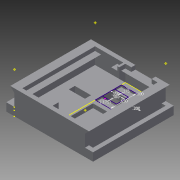
# Autodesk Inventor part: nano_enclosure_v3
Saved by Autodesk Inventor 2015 (Build 190159000, 159)
## iProperties
Created: 2015-03-02
Part Number: nano_enclosure_v3
Material: Generic
Document SubType Name: Modeling
Designer: Jeff
Density: 1 g/cm^3
Appearance: Default
Author: Jeff
Autodesk Inventor part; units mm, degrees
ref_plane "YZ Plane" through (0, 0, 0) normal (1, 0, 0) x (0, 1, 0)
ref_plane "XZ Plane" through (0, 0, 0) normal (0, 1, 0) x (-1, 0, 0)
ref_plane "XY Plane" through (0, 0, 0) normal (0, 0, 1) x (1, 0, 0)
sketch "Sketch2" plane through (0, 0, 0) normal (0, 0, 1) x (1, 0, 0)
  line L0 (0, 0) -> (44.45, 0)
  line L1 (44.45, 0) -> (44.45, 50.8)
  line L2 (44.45, 50.8) -> (0, 50.8)
  line L3 (0, 50.8) -> (0, 0)
  dimension "d0" = 50.8
  dimension "d1" = 44.45
  constraints: 8 end point, 2 parallel, 1 horizontal, 1 perpendicular
  measures "d0" distance of L0.end L1.end
  measures "d1" distance of L1.end L2.end
extrude "Extrusion1" add sketch "Sketch2" along normal blind 25.4
sketch "Sketch3" plane through (0, 0, 25.4) normal (0, 0, 1) x (1, 0, 0)
  line L0 (2.54, 2.54) -> (20.32, 2.54)
  line L1 (20.32, 2.54) -> (20.32, 48.26)
  line L2 (20.32, 48.26) -> (2.54, 48.26)
  line L3 (2.54, 48.26) -> (2.54, 2.54)
  line L4 (0, 0) -> (44.45, 0) projected
  line L5 (0, 50.8) -> (0, 0) projected
  line L6 (44.45, 50.8) -> (0, 50.8) projected
  line L7 (21.59, 2.54) -> (41.91, 2.54)
  line L8 (41.91, 2.54) -> (41.91, 48.26)
  line L9 (41.91, 48.26) -> (21.59, 48.26)
  line L10 (21.59, 48.26) -> (21.59, 2.54)
  line L11 (44.45, 0) -> (44.45, 50.8) projected
  dimension "d4" = 2.54
  dimension "d5" = 2.54
  dimension "d6" = 2.54
  dimension "d7" = 20.32
  dimension "d8" = 2.54
  dimension "d9" = 2.54
  dimension "d10" = 2.54
  dimension "d11" = 22.86
  constraints: 16 end point, 4 parallel, 2 horizontal, 2 perpendicular
  measures "d4" distance between parallel lines of L4 L0
  measures "d5" distance between parallel lines of L5 L3
  measures "d6" distance between parallel lines of L6 L2
  measures "d7" distance between parallel lines of L5 L1
  measures "d8" distance between parallel lines of L4 L7
  measures "d9" distance between parallel lines of L11 L8
  measures "d10" distance between parallel lines of L6 L9
  measures "d11" distance between parallel lines of L11 L10
extrude "Extrusion2" cut sketch "Sketch3" against normal blind 20.32 contours L3 L2 L1 L0 | L10 L9 L8 L7
sketch "Sketch4" plane through (0, 0, 0) normal (0, 0, -1) x (-1, 0, 0)
  circle A0 centre (-12.7, 17.78) radius 8.89
  line L0 (0, 50.8) -> (0, 0) projected
  line L1 (0, 0) -> (-44.45, 0) projected
  dimension "d14" = 17.78
  dimension "d17" = 12.7
  dimension "d18" = 17.78
  constraints: 1 centre point
  measures "d14" diameter of A0
  measures "d17" distance from line of L0 A0.centre
  measures "d18" distance from line of L1 A0.centre
extrude "Extrusion3" cut sketch "Sketch4" against normal blind 3.175
sketch "Sketch5" plane through (0, 0, 0) normal (0, 0, -1) x (-1, 0, 0)
  point P0 (0, 0)
sketch "Sketch6" plane through (12.7, 17.78, 3.175) normal (0, 0, -1) x (-1, 0, 0)
  circle A0 centre (0, 0) radius 8.89 projected
  line L0 (0, 0) -> (-5.08, 0)
  line L1 (-5.08, 0) -> (-5.08, 12.7)
  line L2 (-5.08, 12.7) -> (0, 12.7)
  line L3 (0, 12.7) -> (0, 0)
  line L4 (0, 0) -> (5.08, 0)
  line L5 (5.08, 0) -> (5.08, 12.7)
  line L6 (5.08, 12.7) -> (0, 12.7)
  line L7 (0, 12.7) -> (0, 0)
  point P0 (12.7, -17.78)
  dimension "d21" = 12.7
  dimension "d22" = 5.08
  dimension "d23" = 5.08
  constraints: 16 end point, 4 parallel, 2 horizontal, 2 perpendicular, 1 point on line
  measures "d21" distance between parallel lines of L4 L6
  measures "d22" distance of L0.start L0.end
  measures "d23" distance between parallel lines of L3 L5
extrude "Extrusion4" cut sketch "Sketch6" along normal blind 5.08 contours L5 L4 L3 A0 | A0 L3 L6 L5 | L1 L2 L3 A0 | A0 L3 L0 L1
sketch "Sketch7" plane through (0, 0, 3.175) normal (0, 0, -1) x (-1, 0, 0)
  point P0 (0, 0)
sketch "Sketch8" plane through (0, 0, 3.175) normal (0, 0, -1) x (-1, 0, 0)
  line L0 (-7.62, 25.0756) -> (-7.62, 30.48) projected
  line L1 (-17.78, 30.48) -> (-7.62, 30.48)
  line L2 (-7.62, 30.48) -> (-7.62, 26.67)
  line L3 (-7.62, 26.67) -> (-17.78, 26.67)
  line L4 (-17.78, 26.67) -> (-17.78, 30.48)
  point P0 (0, 0)
  dimension "d26" = 3.81
  constraints: 8 end point, 2 parallel, 1 horizontal, 1 perpendicular, 1 point on line
  measures "d26" distance between parallel lines of L1 L3
extrude "Extrusion5" cut sketch "Sketch8" against normal blind 2.54
sketch "Sketch14" plane through (41.91, 2.54, 25.4) normal (-1, 0, 0) x (0, 0, 1)
  line L0 (0, 0) -> (-20.32, 0) projected
  line L1 (0, 45.72) -> (-20.32, 45.72) projected
  line L2 (-12.7, 45.72) -> (-12.7, 43.18)
  line L3 (-12.7, 43.18) -> (-15.24, 45.72)
  line L4 (-12.7, 0) -> (-12.7, 2.54)
  line L5 (-12.7, 2.54) -> (-15.24, 0)
  point P0 (-25.4, -2.54)
  dimension "d52" = 45
  dimension "d53" = 2.54
  dimension "d54" = 2.54
  dimension "d55" = 45
  dimension "d56" = 5.08
  dimension "d57" = 5.08
  constraints: 8 end point, 4 point on line, 1 perpendicular, 1 vertical
  measures "d52" angle of L3 L2
  measures "d53" distance of L2.start L2.end
  measures "d54" distance of L4.start L4.end
  measures "d55" angle of L5 L4
  measures "d56" distance of L0.end L5.end
  measures "d57" distance of L1.end L3.end
extrude "Arduino Holder" add sketch "Sketch14" along normal blind 20.32
sketch "Sketch16" plane through (2.54, 2.54, 25.4) normal (0, 1, 0) x (1, 0, 0)
  line L0 (0, 12.7) -> (3.81, 12.7)
  line L1 (3.81, 12.7) -> (0, 16.51)
  line L2 (0, 0) -> (0, 20.32) projected
  line L3 (17.78, 5.08) -> (17.78, 20.32)
  line L4 (17.78, 16.51) -> (13.97, 12.7)
  line L5 (13.97, 12.7) -> (17.78, 12.7)
  line L6 (17.78, 20.32) -> (0, 20.32) projected
  point P0 (-2.54, 25.4)
  dimension "d60" = 45
  dimension "d61" = 3.81
  dimension "d62" = 3.81
  dimension "d64" = 45
  dimension "d144" = 7.62
  dimension "d145" = 7.62
  constraints: 10 end point, 3 point on line, 1 horizontal, 1 midpoint, 1 parallel
  measures "d60" angle of L4 L5
  measures "d61" distance of L4.end L5.end
  measures "d62" distance of L0.start L0.end
  measures "d64" angle of L1 L0
  measures "d144" distance between parallel lines of L6 L5
  measures "d145" distance between parallel lines of L6 L0
extrude "Bluetooth Holder" add sketch "Sketch16" along normal blind 45.72
sketch "Sketch17" plane through (0, 0, 0) normal (-1, 0, 0) x (0, 0, 1)
  line L0 (0, 50.8) -> (25.4, 50.8) projected
  line L1 (0, 0) -> (5.08, 0)
  line L2 (5.08, 0) -> (5.08, 50.8)
  line L3 (5.08, 50.8) -> (0, 50.8)
  line L4 (0, 50.8) -> (0, 0)
  dimension "d68" = 5.08
  constraints: 8 end point, 2 parallel, 1 horizontal, 1 perpendicular, 1 point on line
  measures "d68" distance between parallel lines of L4 L2
extrude "Extrusion13" add sketch "Sketch17" along normal blind 5.08
sketch "Sketch18" plane through (0, 0, 5.08) normal (0, 0, 1) x (1, 0, 0)
  line L0 (0, 50.8) -> (0, 0) projected
  line L1 (0, 2.54) -> (-2.54, 2.54)
  line L2 (-2.54, 2.54) -> (-2.54, 48.26)
  line L3 (-2.54, 48.26) -> (0, 48.26)
  line L4 (0, 48.26) -> (0, 2.54)
  line L5 (0, 50.8) -> (-5.08, 50.8) projected
  line L6 (0, 0) -> (-5.08, 0) projected
  dimension "d71" = 2.54
  dimension "d72" = 2.54
  dimension "d73" = 2.54
  constraints: 8 end point, 2 parallel, 1 horizontal, 1 perpendicular, 1 point on line
  measures "d71" distance of L2.end L3.end
  measures "d72" distance between parallel lines of L5 L3
  measures "d73" distance between parallel lines of L6 L1
extrude "Extrusion14" cut sketch "Sketch18" against normal blind 5.08
sketch "Sketch19" plane through (44.45, 0, 0) normal (1, 0, 0) x (0, 0, -1)
  line L0 (0, 50.8) -> (-25.4, 50.8) projected
  line L1 (0, 0) -> (-5.08, 0)
  line L2 (-5.08, 0) -> (-5.08, 50.8)
  line L3 (-5.08, 50.8) -> (0, 50.8)
  line L4 (0, 50.8) -> (0, 0)
  dimension "d76" = 5.08
  constraints: 8 end point, 2 parallel, 1 horizontal, 1 perpendicular, 1 point on line
  measures "d76" distance between parallel lines of L4 L2
extrude "Extrusion15" add sketch "Sketch19" along normal blind 5.08
sketch "Sketch21" plane through (44.45, 0, 5.08) normal (0, 0, 1) x (1, 0, 0)
  line L0 (0, 0) -> (0, 50.8) projected
  line L1 (0, 2.54) -> (2.54, 2.54)
  line L2 (2.54, 2.54) -> (2.54, 48.26)
  line L3 (2.54, 48.26) -> (0, 48.26)
  line L4 (0, 48.26) -> (0, 2.54)
  line L5 (0, 50.8) -> (5.08, 50.8) projected
  line L6 (0, 0) -> (5.08, 0) projected
  line L7 (5.08, 50.8) -> (5.08, 0) projected
  point P0 (-44.45, 0)
  dimension "d79" = 2.54
  dimension "d81" = 2.54
  dimension "d82" = 2.54
  constraints: 8 end point, 2 parallel, 1 horizontal, 1 perpendicular, 1 point on line
  measures "d79" distance between parallel lines of L5 L3
  measures "d81" distance between parallel lines of L6 L1
  measures "d82" distance between parallel lines of L7 L2
extrude "Extrusion16" cut sketch "Sketch21" against normal blind 5.08 contours L0 L3 L2 L1
sketch "Sketch28" plane through (0, 0, 25.4) normal (-1, 0, 0) x (0, 0, 1)
  line L0 (-20.32, 0) -> (0, 0) projected
  line L1 (0, 50.8) -> (-10.16, 50.8)
  line L2 (-10.16, 50.8) -> (-10.16, 0)
  line L3 (-10.16, 0) -> (0, 0)
  line L4 (0, 0) -> (0, 50.8)
  point P0 (-25.4, 0)
  dimension "d141" = 10.16
  constraints: 8 end point, 2 parallel, 1 horizontal, 1 midpoint, 1 perpendicular
  measures "d141" distance between parallel lines of L2 L4
extrude "Height Reduce" cut sketch "Sketch28" against normal blind 48.26
sketch "Sketch30" plane through (0, 0, 5.08) normal (0, 0, 1) x (1, 0, 0)
  line L0 (22.86, 5.08) -> (40.64, 5.08)
  line L1 (40.64, 5.08) -> (40.64, 26.67)
  line L2 (40.64, 26.67) -> (22.86, 26.67)
  line L3 (22.86, 26.67) -> (22.86, 5.08)
  line L4 (21.59, 2.54) -> (21.59, 48.26) projected
  line L5 (41.91, 48.26) -> (41.91, 2.54) projected
  line L6 (41.91, 2.54) -> (21.59, 2.54) projected
  point P0 (0, 0)
  point P1 (24.13, 12.7)
  point P2 (44.45, 30.48)
  dimension "d146" = 1.27
  dimension "d147" = 1.27
  dimension "d148" = 21.59
  dimension "d149" = 2.54
  dimension "d150" = 17.78
  constraints: 8 end point, 2 parallel, 1 horizontal, 1 perpendicular, 2 other
  measures "d148" distance between parallel lines of L2 L0
  measures "d149" distance between parallel lines of L6 L0
  measures "d150" distance between parallel lines of L3 L1
extrude "Extrusion27" cut sketch "Sketch30" against normal blind 2.54
sketch "Sketch31" plane through (0, 0, 5.08) normal (0, 0, 1) x (1, 0, 0)
  line L0 (21.59, 2.54) -> (21.59, 48.26) projected
  line L1 (41.91, 48.26) -> (41.91, 2.54) projected
  line L2 (21.59, 45.72) -> (41.91, 45.72)
  line L3 (41.91, 45.72) -> (41.91, 29.21)
  line L4 (41.91, 29.21) -> (21.59, 29.21)
  line L5 (21.59, 29.21) -> (21.59, 45.72)
  line L6 (21.59, 48.26) -> (41.91, 48.26) projected
  line L7 (21.59, 41.275) -> (30.48, 41.275)
  line L8 (30.48, 41.275) -> (30.48, 33.655)
  line L9 (30.48, 33.655) -> (21.59, 33.655)
  line L10 (21.59, 33.655) -> (21.59, 41.275)
  line L11 (41.91, 45.72) -> (36.83, 45.72)
  line L12 (36.83, 45.72) -> (36.83, 29.21)
  line L13 (36.83, 29.21) -> (41.91, 29.21)
  line L14 (41.91, 29.21) -> (41.91, 45.72)
  point P0 (0, 0)
  point P1 (24.13, 33.02)
  dimension "d157" = 2.54
  dimension "d158" = 16.51
  dimension "d159" = 4.445
  dimension "d160" = 7.62
  dimension "d161" = 8.89
  dimension "d162" = 4.445
  dimension "d163" = 5.08
  constraints: 24 end point, 6 parallel, 3 horizontal, 3 perpendicular, 3 point on line, 2 other
  measures "d157" distance between parallel lines of L2 L6
  measures "d158" distance between parallel lines of L4 L2
  measures "d159" distance between parallel lines of L7 L2
  measures "d160" distance between parallel lines of L9 L7
  measures "d161" distance between parallel lines of L8 L10
  measures "d162" distance between parallel lines of L4 L9
  measures "d163" distance between parallel lines of L1 L12
extrude "Extrusion28" cut sketch "Sketch31" against normal blind 25.4 contours L0 L7 L8 L9
extrude "Extrusion29" cut sketch "Sketch31" against normal blind 2.54 contours L12 L2 L1 L4
extrude "Extrusion30" cut sketch "Sketch31" against normal blind 1.27 contours L0 L9 L8 L7 L2 L12 L4
sketch "Sketch33" plane through (44.45, 2.54, 0) normal (1, 0, 0) x (0, 0, -1)
  line L0 (-5.08, 48.26) -> (-15.24, 48.26) projected
  line L1 (-15.24, -2.54) -> (-12.7, -2.54)
  line L2 (-12.7, -2.54) -> (-12.7, 48.26)
  line L3 (-12.7, 48.26) -> (-15.24, 48.26)
  line L4 (-15.24, 48.26) -> (-15.24, -2.54)
  point P0 (0, -2.54)
  dimension "d194" = 2.54
  constraints: 8 end point, 2 parallel, 1 horizontal, 1 perpendicular, 1 point on line
  measures "d194" distance between parallel lines of L4 L2
extrude "Extrusion33" add sketch "Sketch33" along normal blind 2.54
sketch "Sketch35" plane through (0, 2.54, 0) normal (-1, 0, 0) x (0, 0, 1)
  line L0 (5.08, 48.26) -> (15.24, 48.26) projected
  line L1 (15.24, -2.54) -> (12.7, -2.54)
  line L2 (12.7, -2.54) -> (12.7, 48.26)
  line L3 (12.7, 48.26) -> (15.24, 48.26)
  line L4 (15.24, 48.26) -> (15.24, -2.54)
  point P0 (0, -2.54)
  dimension "d197" = 2.54
  constraints: 8 end point, 2 parallel, 1 horizontal, 1 perpendicular, 1 point on line
  measures "d197" distance between parallel lines of L2 L4
extrude "Extrusion34" add sketch "Sketch35" along normal blind 2.54
sketch "Sketch36" plane through (-5.08, 0, 5.08) normal (0, -1, 0) x (1, 0, 0)
  line L0 (2.54, 10.16) -> (5.08, 7.62)
  line L1 (5.08, 7.62) -> (2.54, 7.62)
  line L2 (5.08, 7.62) -> (2.54, 7.62) projected
  line L3 (2.54, 7.62) -> (2.54, 10.16)
  line L4 (49.53, 7.62) -> (52.07, 10.16)
  line L5 (52.07, 10.16) -> (52.07, 7.62)
  line L6 (52.07, 7.62) -> (49.53, 7.62)
  point P0 (5.08, -5.08)
  constraints: 12 end point, 3 perpendicular, 2 equal length, 1 point on line
extrude "Extrusion35" cut sketch "Sketch36" against normal blind 50.8
sketch "Sketch37" plane through (-5.08, 50.8, 5.08) normal (0, 1, 0) x (1, 0, 0)
  line L0 (52.07, -10.16) -> (2.54, -10.16) projected
  line L1 (43.18, -10.16) -> (30.48, -10.16)
  line L2 (30.48, -10.16) -> (30.48, -7.62)
  line L3 (30.48, -7.62) -> (43.18, -7.62)
  line L4 (43.18, -7.62) -> (43.18, -10.16)
  line L5 (26.67, -10.16) -> (26.67, -7.62) projected
  line L6 (46.99, -10.16) -> (46.99, -7.62) projected
  point P0 (5.08, 5.08)
  dimension "d202" = 2.54
  dimension "d203" = 12.7
  dimension "d204" = 3.81
  dimension "d205" = 3.81
  constraints: 8 end point, 2 parallel, 1 horizontal, 1 perpendicular, 1 point on line
  measures "d202" distance between parallel lines of L3 L0
  measures "d203" distance between parallel lines of L4 L2
  measures "d204" distance between parallel lines of L5 L2
  measures "d205" distance between parallel lines of L6 L4
extrude "USB hole" cut sketch "Sketch37" against normal blind 2.54
sketch "Sketch38" plane through (20.32, 2.54, 5.08) normal (-1, 0, 0) x (0, 0, 1)
  line L0 (0, 0) -> (3.81, 3.81)
  line L1 (3.81, 3.81) -> (3.81, 41.91)
  line L2 (3.81, 41.91) -> (0, 45.72)
  line L3 (0, 45.72) -> (0, 0)
  line L4 (3.81, 3.81) -> (10.16, 3.81)
  line L5 (10.16, 3.81) -> (10.16, 41.91)
  line L6 (10.16, 0) -> (10.16, 45.72) projected
  line L7 (10.16, 41.91) -> (3.81, 41.91)
  point P0 (-5.08, -2.54)
  dimension "d209" = 3.81
  dimension "d210" = 135
  dimension "d211" = 135
  constraints: 14 end point, 1 collinear, 1 horizontal, 1 parallel, 1 perpendicular, 1 point on line, 1 vertical
  measures "d209" distance between parallel lines of L3 L1
  measures "d210" angle of L0 L1
  measures "d211" angle of L1 L2
extrude "Center column remove" cut sketch "Sketch38" along normal mid plane 7.62
body "Solid1"
